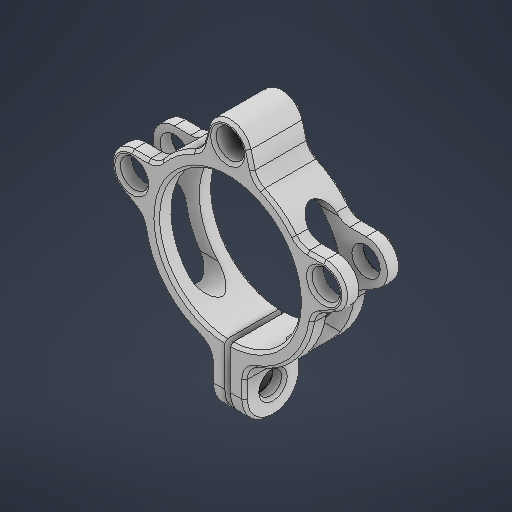
# Autodesk Inventor part: Day02_Task04
Saved by Autodesk Inventor 2027.1 (Build 311270010, 270A)
## iProperties
Created: 2026-08-06
Part Number: Day02_Task04
Material: 일반
Document SubType Name: Modeling
Designer: lkh06
Density: 1 g/cm^3
Appearance: 기본값
Author: lkh06
Autodesk Inventor part; units mm, degrees
ref_plane "YZ Plane" through (0, 0, 0) normal (1, 0, 0) x (0, 1, 0)
ref_plane "XZ Plane" through (0, 0, 0) normal (0, 1, 0) x (-1, 0, 0)
ref_plane "XY Plane" through (0, 0, 0) normal (0, 0, 1) x (1, 0, 0)
sketch "스케치1" plane through (0, 0, 0) normal (0, 0, 1) x (1, 0, 0)
  arc A0 (1, -24.98) -> (-1, -24.98) centre (0, 0) ccw
  line L0 (0, 0) -> (0, -50) construction
  line L1 (1, -50) -> (1, -24.98)
  line L2 (-1, -50) -> (-1, -24.98)
  line L3 (1, -50) -> (6, -50)
  line L4 (6, -50) -> (6, -33.9411)
  line L5 (-1, -50) -> (-6, -50)
  line L6 (-6, -50) -> (-6, -33.9411)
  arc A1 (10, -28.2843) -> (6, -33.9411) centre (12, -33.9411) ccw
  arc A2 (-6, -33.9411) -> (-10, -28.2843) centre (-12, -33.9411) ccw
  line L7 (0, 0) -> (0, 35) construction
  circle A3 centre (0, 35) radius 5
  arc A4 (7.2444, 36.9411) -> (-7.2444, 36.9411) centre (0, 35) ccw
  arc A5 (-12.1073, 27.4484) -> (-8.7332, 31.3852) centre (-14.5287, 32.9381) ccw
  arc A6 (8.7332, 31.3852) -> (12.1073, 27.4484) centre (14.5287, 32.9381) ccw
  line L8 (-7.2444, 36.9411) -> (-8.7332, 31.3852)
  line L9 (7.2444, 36.9411) -> (8.7332, 31.3852)
  line L10 (0, 0) -> (33.8074, 9.0587) construction
  line L11 (0, 0) -> (35, 0) construction
  circle A7 centre (33.8074, 9.0587) radius 5
  arc A8 (37.5574, 2.5635) -> (33.8074, 16.5587) centre (33.8074, 9.0587) ccw
  line L12 (33.8074, 16.5587) -> (28.0554, 16.5587)
  line L13 (37.5574, 2.5635) -> (32.576, -0.3125)
  arc A9 (10, -28.2843) -> (29.6467, -4.5906) centre (0, 0) ccw
  arc A10 (23.3795, 18.7989) -> (12.1073, 27.4484) centre (0, 0) ccw
  arc A11 (23.3795, 18.7989) -> (28.0554, 16.5587) centre (28.0554, 22.5587) ccw
  arc A12 (32.576, -0.3125) -> (29.6467, -4.5906) centre (35.576, -5.5087) ccw
  circle A13 centre (-33.8074, 9.0587) radius 5
  arc A14 (-33.8074, 16.5587) -> (-37.5574, 2.5635) centre (-33.8074, 9.0587) ccw
  line L14 (-33.8074, 16.5587) -> (-28.0554, 16.5587)
  line L15 (-37.5574, 2.5635) -> (-32.576, -0.3125)
  arc A15 (-28.0554, 16.5587) -> (-23.3795, 18.7989) centre (-28.0554, 22.5587) ccw
  arc A16 (-29.6467, -4.5906) -> (-32.576, -0.3125) centre (-35.576, -5.5087) ccw
  arc A17 (-12.1073, 27.4484) -> (-23.3795, 18.7989) centre (0, 0) ccw
  arc A18 (-29.6467, -4.5906) -> (-10, -28.2843) centre (0, 0) ccw
  line L16 (-41.3074, 9.0587) -> (41.3074, 9.0587) construction
  line L17 (0, 0) -> (-41.3074, 0) construction
  point P0 (-6, -41.9706)
  point P1 (-35, 0)
  dimension "d0" = 50
  dimension "d10" = 6
  dimension "d13" = 2
  dimension "d15" = 5
  dimension "d16" = 12
  dimension "d19" = 50
  dimension "d20" = 1
  dimension "d21" = 35
  dimension "d23" = 10
  dimension "d24" = 15
  dimension "d28" = 30
  dimension "d30" = 35
  dimension "d31" = 15
  dimension "d34" = 30
  dimension "d37" = 30
  dimension "d39" = 82.6148
  dimension "d40" = 41.3074
  constraints: 36 end point, 34 point on circle, 19 centre point, 15 tangent, 12 symmetric about line, 8 coincident, 8 equal radius, 4 equal length, 4 horizontal, 3 vertical, 2 perpendicular, 1 midpoint, 1 parallel, 1 point on line, 6 other
  measures "d0" diameter of A0
  measures "d10" radius of A2
  measures "d13" distance between parallel lines of L1 L2
  measures "d15" distance from line of L2 point (-6, -41.971)
  measures "d16" distance between parallel lines of L4 L6
  measures "d19" distance from line of L5 point (0, 0)
  measures "d20" distance from line of L1 point (0, 0)
  measures "d21" distance of L0.start L7.end
  measures "d23" diameter of A3
  measures "d24" diameter of A4
  measures "d28" angle of L9 L8
  measures "d30" distance of L0.start L10.end
  measures "d31" angle of L11 L10
  measures "d34" angle of L13 L12
  measures "d37" radius of A18
  measures "d39" distance of L16.start L16.end
  measures "d40" distance of L0.start L17.end
sketch "스케치12" plane through (0, 0, 0) normal (1, 0, 0) x (0, 1, 0)
  line L0 (0, 10) -> (0, -10)
  line L1 (42.1562, 0) -> (-50.3261, 0)
  line L2 (42.5001, -10) -> (-49.9822, -10)
  line L3 (-49.9822, -10) -> (-49.9822, 10)
  line L4 (-49.9822, 10) -> (42.5001, 10)
  line L5 (42.5001, 10) -> (42.5001, -10)
  arc A0 (-39.9822, 10) -> (-39.9822, -10) centre (-39.9822, 0) ccw
  circle A1 centre (-39.9822, 0) radius 4
  arc A2 (-16.9822, 5) -> (-16.9822, -5) centre (-16.9822, 0) ccw
  arc A3 (18.0178, -5) -> (18.0178, 5) centre (18.0178, 0) ccw
  line L6 (18.0178, -5) -> (-16.9822, -5)
  line L7 (18.0178, 5) -> (-16.9822, 5)
  point P0 (0, 0)
  point P1 (42.5001, 0)
  point P2 (0, 0)
  dimension "d85" = 20
  dimension "d89" = 49.9822
  dimension "d90" = 42.5001
  dimension "d91" = 10
  dimension "d93" = 8
  dimension "d94" = 10
  dimension "d95" = 23
  dimension "d96" = 10
  dimension "d97" = 35
  constraints: 16 end point, 7 tangent, 6 point on circle, 5 point on line, 4 centre point, 2 horizontal, 2 midpoint, 2 parallel, 1 coincident, 1 perpendicular
  measures "d85" distance of L4.end L2.start
  measures "d89" horizontal distance of L2.end point (0, 0)
  measures "d90" horizontal distance of L2.start point (0, 0)
  measures "d91" vertical distance of L2.start point (0, 0)
  measures "d93" diameter of A1
  measures "d94" diameter of A2
  measures "d95" distance of A0.centre A2.centre
  measures "d96" diameter of A3
  measures "d97" distance of A2.centre A3.centre
extrude "돌출3" add sketch "스케치1" along normal mid plane 20
extrude "돌출4" cut sketch "스케치12" along normal mid plane 300 contours L4 L5 L2 L0 L6 A3 L7 | L0 L7 A2 L1 A1 A0 L4 | L1 A1 A2 L6 L0 L2 A0 keep common part
chamfer "모따기3" distance 1 angle 45 56 edges at (0, 25, 10) (-38.8074, 9.0587, 10) (-9.973, 29.0335, 10) (-18.2628, 23.8006, 10) (-25.463, 17.1476, 10) (-30.9314, 16.5587, 10) (-41.0518, 10.9998, 10) (-35.0667, 1.1255, 10) (-30.6254, -2.1188, 10) (-23.0936, -19.1491, 10) (-7.101, -30.477, 10) (-6, -36.9617, 10) (-6, -49.9822, 0) (-6, -36.9617, -10) (-7.101, -30.477, -10) (-23.0936, -19.1491, -10) (-30.6254, -2.1188, -10) (-35.0667, 1.1255, -10) (-41.0518, 10.9998, -10) (-30.9314, 16.5587, -10) (-25.463, 17.1476, -10) (-18.2628, 23.8006, -10) (-9.973, 29.0335, -10) (-7.9888, 34.1631, -10) (0, 42.5, -10) (7.9888, 34.1631, -10) (9.973, 29.0335, -10) (18.2628, 23.8006, -10) (25.463, 17.1476, -10) (30.9314, 16.5587, -10) (41.0518, 10.9998, -10) (35.0667, 1.1255, -10) (30.6254, -2.1188, -10) (23.0936, -19.1491, -10) (7.101, -30.477, -10) (6, -36.9617, -10) (6, -49.9822, 0) (6, -36.9617, 10) (7.101, -30.477, 10) (23.0936, -19.1491, 10) (30.6254, -2.1188, 10) (35.0667, 1.1255, 10) (41.0518, 10.9998, 10) (30.9314, 16.5587, 10) (25.463, 17.1476, 10) (18.2628, 23.8006, 10) (9.973, 29.0335, 10) (7.9888, 34.1631, 10) (0, 42.5, 10) (-7.9888, 34.1631, 10) (-5, 35, 10) (28.8074, 9.0587, 10) (6, -43.9822, 0) (1, -43.9822, 0) (-1, -43.9822, 0) (-6, -43.9822, 0)
chamfer "모따기4" distance 1 angle 45 4 edges at (0, 25, -10) (28.8074, 9.0587, -10) (-38.8074, 9.0587, -10) (-5, 35, -10)
